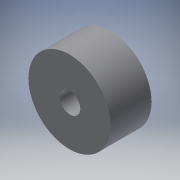
# Autodesk Inventor part: wheel
Saved by Autodesk Inventor 2019 (Build 230136000, 136)
## iProperties
Created: 2020-03-03
Part Number: wheel
Material: Generic
Document SubType Name: Modeling
Designer: Hp
Density: 1 g/cm^3
Appearance: Default
Author: Hp
Autodesk Inventor part; units mm, degrees
ref_plane "YZ Plane" through (0, 0, 0) normal (1, 0, 0) x (0, 1, 0)
ref_plane "XZ Plane" through (0, 0, 0) normal (0, 1, 0) x (-1, 0, 0)
ref_plane "XY Plane" through (0, 0, 0) normal (0, 0, 1) x (1, 0, 0)
sketch "Sketch1" plane through (0, 0, 0) normal (0, 0, 1) x (1, 0, 0)
  circle A0 centre (0, 0) radius 20
  dimension "d0" = 40
  constraints: 1 centre point, 1 coincident
  measures "d0" diameter of A0
extrude "Extrusion1" add sketch "Sketch1" along normal blind 20
sketch "Sketch2" plane through (0, 0, 20) normal (0, 0, 1) x (1, 0, 0)
  point P0 (0, 0)
  point P1 (0.2579, -0.3016)
hole "Hole1" at (0.2579, -0.3016, 20) direction (0, 0, -1) diameter 10 depth 30 tip angle 118
body "Solid1"
